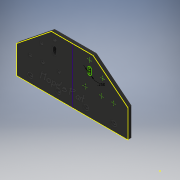
# Autodesk Inventor part: Junk Part
Saved by Autodesk Inventor 2017 (Build 210142000, 142)
## iProperties
Created: 2017-05-17
Part Number: Junk Part
Material: Rubber
Document SubType Name: Modeling
Designer: User
Density: 0.93 g/cm^3
Appearance: Rubber - Black
Mass: 100.023 g
Surface Area: 393.354 cm^2
Volume: 107.552 cm^3
Author: User
Autodesk Inventor part; units mm, degrees
ref_plane "XZ Plane" through (0, 0, 0) normal (0, 1, 0) x (-1, 0, 0)
ref_plane "XY Plane" through (0, 0, 0) normal (0, 0, 1) x (1, 0, 0)
sketch "Sketch1" plane through (0, 0, 0) normal (0, 0, 1) x (1, 0, 0)
  line L0 (-262.1103, 19.715) -> (-58.9103, 19.715)
  line L1 (-58.9103, 19.715) -> (-58.9103, 70.515)
  line L2 (-58.9103, 70.515) -> (-122.4103, 121.315)
  line L3 (-122.4103, 121.315) -> (-198.6103, 121.315)
  line L4 (-198.6103, 121.315) -> (-262.1103, 70.515)
  line L5 (-262.1103, 70.515) -> (-262.1103, 19.715)
  point P0 (0, 0)
  dimension "d0" = 203.2
  dimension "d1" = 50.8
  dimension "d2" = 50.8
  dimension "d3" = 101.6
  dimension "d4" = 76.2
  dimension "d5" = 63.5
  constraints: 12 end point, 2 parallel, 1 horizontal, 1 perpendicular
  measures "d0" distance of L0.start L0.end
  measures "d1" distance of L4.end L0.start
  measures "d2" distance of L0.end L1.end
  measures "d3" distance between parallel lines of L0 L3
  measures "d4" distance of L2.end L3.end
  measures "d5" distance from line of L2.end L1
extrude "Extrusion1" add sketch "Sketch1" along normal blind 6.35
sketch "Sketch2" plane through (0, 0, 6.35) normal (0, 0, 1) x (1, 0, 0)
  line L0 (-262.1103, 19.715) -> (-58.9103, 19.715) projected
  line L1 (-58.9103, 19.715) -> (-58.9103, 70.515) projected
  line L2 (-58.9103, 70.515) -> (-122.4103, 121.315) projected
  line L3 (-122.4103, 121.315) -> (-198.6103, 121.315) projected
  line L4 (-198.6103, 121.315) -> (-262.1103, 70.515) projected
  line L5 (-262.1103, 70.515) -> (-262.1103, 19.715) projected
  point P0 (0, 0)
  point P1 (-84.3103, 32.415)
  dimension "d8" = 12.7
  dimension "d9" = 25.4
  measures "d8" distance from line of point (-84.31, 32.415) L0
  measures "d9" distance from line of point (-84.31, 32.415) L1
hole "Hole1" at (-84.3103, 32.415, 6.35) direction (0, 0, -1) diameter 4.9784 depth 19.05 tip angle 118 counterbore diameter 9.525 counterbore depth 1.27 thread size "1/4-20 UNC" class "2B" standard "ANSI Unified Screw Threads"
pattern_linear "Rectangular Pattern1" count 4 spacing 50.8 along (-1, 0, 0) of "Hole1"
sketch "Sketch3" plane through (0, 0, 6.35) normal (0, 0, 1) x (1, 0, 0)
  line L0 (-262.1103, 19.715) -> (-58.9103, 19.715) projected
  line L1 (-58.9103, 19.715) -> (-58.9103, 70.515) projected
  line L2 (-58.9103, 70.515) -> (-122.4103, 121.315) projected
  line L3 (-122.4103, 121.315) -> (-198.6103, 121.315) projected
  line L4 (-198.6103, 121.315) -> (-262.1103, 70.515) projected
  line L5 (-262.1103, 70.515) -> (-262.1103, 19.715) projected
  line L6 (-128.7603, 100.9956) -> (-128.7603, 86.3997) construction
  line L7 (-131.9353, 97.8206) -> (-131.9353, 89.5747)
  line L8 (-125.5853, 89.5747) -> (-125.5853, 97.8206)
  arc A0 (-125.5853, 97.8206) -> (-131.9353, 97.8206) centre (-128.7603, 97.8206) ccw
  arc A1 (-131.9353, 89.5747) -> (-125.5853, 89.5747) centre (-128.7603, 89.5747) ccw
  point P0 (0, 0)
  point P1 (-128.7603, 93.6976)
  point P2 (-136.9971, 64.7412)
  point P3 (-107.099, 64.7412)
  point P4 (-84.3103, 64.7412)
  point P5 (-128.7603, 110.8832)
  point P6 (-104.7448, 93.6976)
  dimension "d20" = 6.35
  constraints: 8 end point, 6 point on circle, 4 tangent, 3 point on line, 2 centre point, 1 midpoint, 1 parallel, 1 vertical
  measures "d20" diameter of A1
hole "Hole2" at (-136.9971, 64.7412, 6.35) at (-107.099, 64.7412, 6.35) at (-84.3103, 64.7412, 6.35) at (-128.7603, 110.8832, 6.35) at (-104.7448, 93.6976, 6.35) direction (0, 0, -1) diameter 4.9784 end through all thread size "1/4-20 UNC" class "2B" standard "ANSI Unified Screw Threads"
extrude "Extrusion2" cut sketch "Sketch3" against normal blind 25.4 contours A0 L8 A1 L7
sketch "Sketch4" plane through (0, 0, 6.35) normal (0, 0, 1) x (1, 0, 0)
  line L0 (-262.1103, 19.715) -> (-58.9103, 19.715) projected
  line L1 (-122.4103, 121.315) -> (-198.6103, 121.315) projected
  line L2 (-160.5103, 121.315) -> (-160.5103, 19.715)
  line L3 (-262.1103, 19.715) -> (-58.9103, 19.715) projected
  point P0 (0, 0)
  constraints: 2 end point, 2 midpoint
ref_plane "Work Plane1" through (-160.5103, 121.315, 6.35) normal (1, 0, 0) x (0, -1, 0)
mirror "Mirror1" about plane through (-160.5103, 121.315, 6.35) normal (1, 0, 0) of "Hole2", "Extrusion2"
sketch "Sketch5" plane through (0, 0, 6.35) normal (0, 0, 1) x (1, 0, 0)
  line L0 (-218.3313, 50.345) -> (-138.1632, 50.345) construction
  line L1 (-138.1632, 50.345) -> (-138.1632, 34.1767) construction
  line L2 (-138.1632, 34.1767) -> (-218.3313, 34.1767) construction
  line L3 (-218.3313, 34.1767) -> (-218.3313, 50.345) construction
  spline S0 degree 2 poles (-207.5694, 47.7336) (-207.9469, 47.652) (-208.6507, 47.4888) knots 0 0 0 1 1 1
  line L4 (-208.6507, 47.4888) -> (-211.1601, 38.1245)
  line L5 (-211.1601, 38.1245) -> (-211.6498, 38.1245)
  line L6 (-211.6498, 38.1245) -> (-209.1302, 47.3868)
  line L7 (-209.1302, 47.3868) -> (-215.8831, 45.8669)
  line L8 (-215.8831, 45.8669) -> (-218.1375, 37.4308)
  line L9 (-218.1375, 37.4308) -> (-218.6271, 37.4308)
  line L10 (-218.6271, 37.4308) -> (-216.3931, 45.7649)
  spline S1 degree 2 poles (-216.3931, 45.7649) (-216.7094, 45.6731) (-217.0358, 45.6118) knots 0 0 0 1 1 1
  line L11 (-217.0358, 45.6118) -> (-217.0358, 46.0811)
  line L12 (-217.0358, 46.0811) -> (-216.2605, 46.2647)
  line L13 (-216.2605, 46.2647) -> (-215.4037, 49.4473)
  line L14 (-215.4037, 49.4473) -> (-214.9242, 49.4473)
  line L15 (-214.9242, 49.4473) -> (-215.7403, 46.3769)
  line L16 (-215.7403, 46.3769) -> (-209.0486, 47.8662)
  line L17 (-209.0486, 47.8662) -> (-208.4263, 50.1308)
  line L18 (-208.4263, 50.1308) -> (-207.9367, 50.1308)
  line L19 (-207.9367, 50.1308) -> (-208.5181, 47.9682)
  line L20 (-208.5181, 47.9682) -> (-207.5694, 48.2029)
  line L21 (-207.5694, 48.2029) -> (-207.5694, 47.7336)
  spline S2 degree 2 poles (-203.8257, 37.645) (-205.0396, 37.645) (-206.8146, 39.3282) (-206.8146, 40.5318) knots 0 0 0 1 2 2 2
  line L22 (-206.8146, 40.5318) -> (-206.8146, 40.542)
  spline S3 degree 2 poles (-206.8146, 40.542) (-206.8146, 42.2762) (-205.3559, 43.4493) knots 0 0 0 1 1 1
  spline S4 degree 2 poles (-205.3559, 43.4493) (-203.9788, 44.551) (-202.1222, 44.551) knots 0 0 0 1 1 1
  spline S5 degree 2 poles (-202.1222, 44.551) (-200.8777, 44.551) (-199.9902, 43.8165) knots 0 0 0 1 1 1
  spline S6 degree 2 poles (-199.9902, 43.8165) (-199.0518, 43.031) (-199.0518, 41.8069) knots 0 0 0 1 1 1
  spline S7 degree 2 poles (-199.0518, 41.8069) (-199.0518, 39.9912) (-200.5513, 38.7773) knots 0 0 0 1 1 1
  spline S8 degree 2 poles (-200.5513, 38.7773) (-201.9692, 37.645) (-203.8257, 37.645) knots 0 0 0 1 1 1
  spline S9 degree 2 poles (-199.5006, 41.8069) (-199.5006, 42.6944) (-200.8063, 44.0103) (-201.7244, 44.0919) knots 0 0 0 1 2 2 2
  spline S10 degree 2 poles (-201.7244, 44.0919) (-203.4993, 44.2347) (-204.8968, 43.2351) knots 0 0 0 1 1 1
  spline S11 degree 2 poles (-204.8968, 43.2351) (-206.3657, 42.1742) (-206.3657, 40.5318) knots 0 0 0 1 1 1
  line L23 (-206.3657, 40.5318) -> (-206.3657, 40.5216)
  spline S12 degree 2 poles (-206.3657, 40.5216) (-206.3657, 39.522) (-204.856, 38.0939) (-203.8257, 38.0939) knots 0 0 0 1 2 2 2
  spline S13 degree 2 poles (-203.8257, 38.0939) (-202.1732, 38.0939) (-200.8777, 39.0935) knots 0 0 0 1 1 1
  spline S14 degree 2 poles (-200.8777, 39.0935) (-199.5006, 40.185) (-199.5006, 41.8069) knots 0 0 0 1 1 1
  spline S15 degree 2 poles (-190.3607, 42.7148) (-190.5341, 40.2972) (-193.2271, 38.8283) knots 0 0 0 1 1 1
  spline S16 degree 2 poles (-193.2271, 38.8283) (-195.1245, 37.7878) (-197.4094, 37.5226) knots 0 0 0 1 1 1
  line L24 (-197.4094, 37.5226) -> (-198.3071, 34.1767)
  line L25 (-198.3071, 34.1767) -> (-198.7865, 34.1767)
  line L26 (-198.7865, 34.1767) -> (-197.8991, 37.4818)
  spline S17 degree 2 poles (-197.8991, 37.4818) (-198.1439, 37.4818) (-198.2153, 37.492) knots 0 0 0 1 1 1
  line L27 (-198.2153, 37.492) -> (-198.1541, 37.9204)
  spline S18 degree 2 poles (-198.1541, 37.9204) (-198.0929, 37.9102) (-197.7869, 37.9408) knots 0 0 0 1 1 1
  line L28 (-197.7869, 37.9408) -> (-196.2261, 43.7451)
  spline S19 degree 2 poles (-196.2261, 43.7451) (-196.3282, 43.7349) (-196.7362, 43.6227) (-196.8382, 43.5921) knots 0 0 0 1 2 2 2
  line L29 (-196.8382, 43.5921) -> (-196.8382, 44.0613)
  spline S20 degree 2 poles (-196.8382, 44.0613) (-196.5628, 44.1429) (-196.0935, 44.2245) knots 0 0 0 1 1 1
  spline S21 degree 2 poles (-196.0935, 44.2245) (-196.0323, 44.4388) (-195.9201, 44.806) knots 0 0 0 1 1 1
  line L30 (-195.9201, 44.806) -> (-195.4509, 44.806)
  line L31 (-195.4509, 44.806) -> (-195.6039, 44.3163)
  spline S22 degree 2 poles (-195.6039, 44.3163) (-194.0228, 44.551) (-193.0333, 44.551) knots 0 0 0 1 1 1
  spline S23 degree 2 poles (-193.0333, 44.551) (-190.2179, 44.551) (-190.3607, 42.7148) knots 0 0 0 1 1 1
  spline S24 degree 2 poles (-190.8095, 42.7352) (-190.6973, 44.1327) (-193.0231, 44.1327) knots 0 0 0 1 1 1
  spline S25 degree 2 poles (-193.0231, 44.1327) (-194.084, 44.1327) (-195.7365, 43.8267) knots 0 0 0 1 1 1
  line L32 (-195.7365, 43.8267) -> (-197.3074, 37.9816)
  spline S26 degree 2 poles (-197.3074, 37.9816) (-195.0939, 38.2877) (-193.4005, 39.2159) knots 0 0 0 1 1 1
  spline S27 degree 2 poles (-193.4005, 39.2159) (-190.9625, 40.5624) (-190.8095, 42.7352) knots 0 0 0 1 1 1
  line L33 (-182.3122, 43.8471) -> (-189.5548, 40.5318)
  spline S28 degree 2 poles (-189.5548, 40.5318) (-189.5854, 40.3788) (-189.5854, 40.2258) knots 0 0 0 1 1 1
  spline S29 degree 2 poles (-189.5854, 40.2258) (-189.616, 39.0425) (-188.851, 38.4203) knots 0 0 0 1 1 1
  spline S30 degree 2 poles (-188.851, 38.4203) (-188.1573, 37.8796) (-187.0046, 37.8796) knots 0 0 0 1 1 1
  spline S31 degree 2 poles (-187.0046, 37.8796) (-185.2705, 37.8796) (-183.9852, 38.8895) knots 0 0 0 1 1 1
  line L34 (-183.9852, 38.8895) -> (-183.6282, 38.5529)
  spline S32 degree 2 poles (-183.6282, 38.5529) (-185.0563, 37.4512) (-186.974, 37.4512) knots 0 0 0 1 1 1
  spline S33 degree 2 poles (-186.974, 37.4512) (-188.3307, 37.4512) (-189.157, 38.1143) knots 0 0 0 1 1 1
  spline S34 degree 2 poles (-189.157, 38.1143) (-190.0955, 38.8487) (-190.0445, 40.2258) knots 0 0 0 1 1 1
  spline S35 degree 2 poles (-190.0445, 40.2258) (-189.9935, 41.6641) (-188.2695, 43.1126) knots 0 0 0 1 1 1
  spline S36 degree 2 poles (-188.2695, 43.1126) (-186.4742, 44.6122) (-184.5564, 44.6122) knots 0 0 0 1 1 1
  spline S37 degree 2 poles (-184.5564, 44.6122) (-183.2813, 44.6122) (-182.3122, 43.8471) knots 0 0 0 1 1 1
  spline S38 degree 2 poles (-183.2507, 43.8879) (-183.8322, 44.2245) (-184.5972, 44.2245) knots 0 0 0 1 1 1
  spline S39 degree 2 poles (-184.5972, 44.2245) (-185.9437, 44.2245) (-188.7898, 42.3068) (-189.3406, 41.1235) knots 0 0 0 1 2 2 2
  line L35 (-189.3406, 41.1235) -> (-183.2507, 43.8879)
  line L36 (-179.9253, 50.1206) -> (-181.0371, 45.4894)
  line L37 (-181.0371, 45.4894) -> (-181.5268, 45.4894)
  line L38 (-181.5268, 45.4894) -> (-180.3843, 50.1206)
  line L39 (-180.3843, 50.1206) -> (-179.9253, 50.1206)
  spline S40 degree 2 poles (-171.1322, 42.3986) (-170.5609, 41.8682) (-170.5609, 41.2969) knots 0 0 0 1 1 1
  spline S41 degree 2 poles (-170.5609, 41.2969) (-170.5609, 39.8688) (-173.611, 38.6141) knots 0 0 0 1 1 1
  spline S42 degree 2 poles (-173.611, 38.6141) (-176.406, 37.4512) (-178.8644, 37.4512) knots 0 0 0 1 1 1
  line L40 (-178.8644, 37.4512) -> (-178.8644, 37.9)
  spline S43 degree 2 poles (-178.8644, 37.9) (-176.5896, 37.9) (-173.8966, 39.0017) knots 0 0 0 1 1 1
  spline S44 degree 2 poles (-173.8966, 39.0017) (-171.0404, 40.1442) (-171.0404, 41.3071) knots 0 0 0 1 1 1
  spline S45 degree 2 poles (-171.0404, 41.3071) (-171.0404, 41.7049) (-171.428, 42.062) knots 0 0 0 1 1 1
  spline S46 degree 2 poles (-171.428, 42.062) (-171.8666, 42.4598) (-172.8051, 42.4598) knots 0 0 0 1 1 1
  spline S47 degree 2 poles (-172.8051, 42.4598) (-173.866, 42.4598) (-175.5695, 41.9294) knots 0 0 0 1 1 1
  spline S48 degree 2 poles (-175.5695, 41.9294) (-176.5284, 41.6029) (-177.5179, 41.2663) knots 0 0 0 1 1 1
  spline S49 degree 2 poles (-177.5179, 41.2663) (-177.5893, 41.2561) (-177.6709, 41.2561) knots 0 0 0 1 1 1
  spline S50 degree 2 poles (-177.6709, 41.2561) (-178.0381, 41.2561) (-178.0381, 41.5621) knots 0 0 0 1 1 1
  spline S51 degree 2 poles (-178.0381, 41.5621) (-178.0381, 41.8069) (-177.7627, 42.1742) knots 0 0 0 1 1 1
  spline S52 degree 2 poles (-177.7627, 42.1742) (-177.0894, 43.0922) (-175.8449, 43.7655) knots 0 0 0 1 1 1
  spline S53 degree 2 poles (-175.8449, 43.7655) (-174.4474, 44.551) (-173.1111, 44.551) knots 0 0 0 1 1 1
  spline S54 degree 2 poles (-173.1111, 44.551) (-172.5909, 44.551) (-172.1114, 44.4286) knots 0 0 0 1 1 1
  line L41 (-172.1114, 44.4286) -> (-172.1114, 44.0001)
  spline S55 degree 2 poles (-172.1114, 44.0001) (-172.5909, 44.1225) (-173.0907, 44.1225) knots 0 0 0 1 1 1
  spline S56 degree 2 poles (-173.0907, 44.1225) (-174.3658, 44.1225) (-175.6613, 43.4187) knots 0 0 0 1 1 1
  spline S57 degree 2 poles (-175.6613, 43.4187) (-176.8038, 42.7862) (-177.4261, 41.9396) knots 0 0 0 1 1 1
  spline S58 degree 2 poles (-177.4261, 41.9396) (-177.6097, 41.6947) (-177.5893, 41.6947) knots 0 0 0 1 1 1
  spline S59 degree 2 poles (-177.5893, 41.6947) (-176.406, 42.0824) (-175.2227, 42.4802) knots 0 0 0 1 1 1
  spline S60 degree 2 poles (-175.2227, 42.4802) (-173.6926, 42.9392) (-172.7541, 42.9392) knots 0 0 0 1 1 1
  spline S61 degree 2 poles (-172.7541, 42.9392) (-171.6932, 42.9392) (-171.1322, 42.3986) knots 0 0 0 1 1 1
  spline S62 degree 2 poles (-154.9333, 48.3865) (-155.7188, 47.1828) (-157.0347, 46.4483) knots 0 0 0 1 1 1
  spline S63 degree 2 poles (-157.0347, 46.4483) (-157.1163, 46.4075) (-159.7379, 45.2242) knots 0 0 0 1 1 1
  spline S64 degree 2 poles (-159.7379, 45.2242) (-160.7069, 44.7856) (-161.7882, 44.5306) knots 0 0 0 1 1 1
  spline S65 degree 2 poles (-161.7882, 44.5306) (-162.7675, 44.3163) (-163.7672, 44.1021) knots 0 0 0 1 1 1
  line L42 (-163.7672, 44.1021) -> (-165.6441, 37.5124)
  line L43 (-165.6441, 37.5124) -> (-166.1542, 37.5124)
  line L44 (-166.1542, 37.5124) -> (-164.2772, 43.9083)
  spline S66 degree 2 poles (-164.2772, 43.9083) (-164.3894, 43.9083) (-165.0321, 43.7553) knots 0 0 0 1 1 1
  line L45 (-165.0321, 43.7553) -> (-165.0321, 44.1939)
  spline S67 degree 2 poles (-165.0321, 44.1939) (-164.6955, 44.3163) (-164.1752, 44.3775) knots 0 0 0 1 1 1
  line L46 (-164.1752, 44.3775) -> (-163.2061, 47.9886)
  spline S68 degree 2 poles (-163.2061, 47.9886) (-163.502, 47.8458) (-164.42, 47.4072) knots 0 0 0 1 1 1
  line L47 (-164.42, 47.4072) -> (-164.42, 47.907)
  spline S69 degree 2 poles (-164.42, 47.907) (-163.9712, 48.1212) (-163.1143, 48.4579) knots 0 0 0 1 1 1
  line L48 (-163.1143, 48.4579) -> (-162.7471, 50.1206)
  line L49 (-162.7471, 50.1206) -> (-162.2575, 50.1206)
  line L50 (-162.2575, 50.1206) -> (-162.5635, 48.6415)
  spline S70 degree 2 poles (-162.5635, 48.6415) (-158.0853, 50.2838) (-155.9738, 50.3144) knots 0 0 0 1 1 1
  spline S71 degree 2 poles (-155.9738, 50.3144) (-154.4743, 50.345) (-154.4743, 49.5188) knots 0 0 0 1 1 1
  spline S72 degree 2 poles (-154.4743, 49.5188) (-154.4743, 49.0699) (-154.9333, 48.3865) knots 0 0 0 1 1 1
  spline S73 degree 2 poles (-155.3413, 48.6517) (-155.0455, 49.0801) (-155.0455, 49.3555) knots 0 0 0 1 1 1
  spline S74 degree 2 poles (-155.0455, 49.3555) (-155.0455, 49.8656) (-155.9942, 49.8656) knots 0 0 0 1 1 1
  spline S75 degree 2 poles (-155.9942, 49.8656) (-157.9833, 49.8656) (-162.6247, 48.0702) knots 0 0 0 1 1 1
  line L51 (-162.6247, 48.0702) -> (-163.6958, 44.5204)
  spline S76 degree 2 poles (-163.6958, 44.5204) (-162.0535, 44.8876) (-161.8392, 44.9488) knots 0 0 0 1 1 1
  spline S77 degree 2 poles (-161.8392, 44.9488) (-160.9008, 45.2038) (-159.9215, 45.6526) knots 0 0 0 1 1 1
  spline S78 degree 2 poles (-159.9215, 45.6526) (-158.6362, 46.2341) (-157.3407, 46.8155) knots 0 0 0 1 1 1
  spline S79 degree 2 poles (-157.3407, 46.8155) (-156.1064, 47.5092) (-155.3413, 48.6517) knots 0 0 0 1 1 1
  line L52 (-147.0685, 43.3983) -> (-148.619, 37.5838)
  line L53 (-148.619, 37.5838) -> (-149.0984, 37.5838)
  line L54 (-149.0984, 37.5838) -> (-148.2314, 40.8175)
  spline S80 degree 2 poles (-148.2314, 40.8175) (-149.9553, 37.7878) (-151.5466, 37.6654) knots 0 0 0 1 1 1
  spline S81 degree 2 poles (-151.5466, 37.6654) (-152.3933, 37.6042) (-153.7602, 38.9201) (-153.7602, 39.7668) knots 0 0 0 1 2 2 2
  spline S82 degree 2 poles (-153.7602, 39.7668) (-153.7602, 39.981) (-153.7092, 40.185) knots 0 0 0 1 1 1
  spline S83 degree 2 poles (-153.7092, 40.185) (-153.2808, 41.8171) (-150.1287, 44.4592) (-148.6496, 44.4592) knots 0 0 0 1 2 2 2
  spline S84 degree 2 poles (-148.6496, 44.4592) (-147.9151, 44.4592) (-147.4051, 44.0715) knots 0 0 0 1 1 1
  line L55 (-147.4051, 44.0715) -> (-147.7315, 43.7553)
  spline S85 degree 2 poles (-147.7315, 43.7553) (-148.16, 44.0715) (-148.7618, 44.0715) knots 0 0 0 1 1 1
  spline S86 degree 2 poles (-148.7618, 44.0715) (-150.0267, 44.0715) (-152.8829, 41.5723) (-153.2604, 40.0728) knots 0 0 0 1 2 2 2
  spline S87 degree 2 poles (-153.2604, 40.0728) (-153.3114, 39.9198) (-153.3114, 39.7668) knots 0 0 0 1 1 1
  spline S88 degree 2 poles (-153.3114, 39.7668) (-153.3114, 39.1139) (-152.2199, 38.0633) (-151.5772, 38.1143) knots 0 0 0 1 2 2 2
  spline S89 degree 2 poles (-151.5772, 38.1143) (-150.6082, 38.1959) (-149.5677, 39.4914) knots 0 0 0 1 1 1
  spline S90 degree 2 poles (-149.5677, 39.4914) (-148.823, 40.4706) (-148.1396, 41.96) knots 0 0 0 1 1 1
  spline S91 degree 2 poles (-148.1396, 41.96) (-147.5887, 43.1739) (-147.5887, 43.3983) knots 0 0 0 1 1 1
  line L56 (-147.5887, 43.3983) -> (-147.0685, 43.3983)
  spline S92 degree 2 poles (-142.6821, 44.1123) (-144.7223, 43.8981) (-145.1201, 42.419) knots 0 0 0 1 1 1
  line L57 (-145.1201, 42.419) -> (-146.4564, 37.4308)
  line L58 (-146.4564, 37.4308) -> (-146.9359, 37.4308)
  line L59 (-146.9359, 37.4308) -> (-145.569, 42.521)
  spline S93 degree 2 poles (-145.569, 42.521) (-145.0997, 44.2857) (-142.6821, 44.5918) knots 0 0 0 1 1 1
  line L60 (-142.6821, 44.5918) -> (-142.6821, 44.1123)
  line L61 (-138.6018, 44.6836) -> (-140.3053, 44.3469)
  line L62 (-140.3053, 44.3469) -> (-142.1619, 37.4308)
  line L63 (-142.1619, 37.4308) -> (-142.6515, 37.4308)
  line L64 (-142.6515, 37.4308) -> (-140.8154, 44.2449)
  line L65 (-140.8154, 44.2449) -> (-142.2435, 43.9593)
  line L66 (-142.2435, 43.9593) -> (-142.2333, 44.4286)
  line L67 (-142.2333, 44.4286) -> (-140.6828, 44.7346)
  line L68 (-140.6828, 44.7346) -> (-139.2343, 50.1308)
  line L69 (-139.2343, 50.1308) -> (-138.7446, 50.1308)
  line L70 (-138.7446, 50.1308) -> (-140.1727, 44.8366)
  line L71 (-140.1727, 44.8366) -> (-138.6018, 45.1528)
  line L72 (-138.6018, 45.1528) -> (-138.6018, 44.6836)
  point P0 (0, 0)
  dimension "d0" = 203.2
  dimension "d1" = 50.8
  dimension "d2" = 50.8
  dimension "d3" = 101.6
  dimension "d4" = 76.2
  dimension "d5" = 63.5
  constraints: 2 other
emboss "Emboss1" sketch "Sketch5" operation cut depth 2.54 direction (0, 0, -1)
equation "\"d2\" = d1"
equation "\"d5\" = -0.5 * d4 + 0.5 * d0"
body "Solid1"
